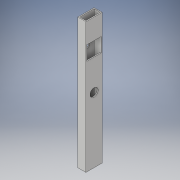
# Autodesk Inventor part: 2x1 16in Aluminum-ver2-1111-2020
Saved by Autodesk Inventor 2018 (Build 220112000, 112)
## iProperties
Created: 2020-01-28
Part Number: 2x1 16in Aluminum-ver2-1111-2020
Material: Generic
Document SubType Name: Modeling
Designer: JMHal
Density: 1 g/cm^3
Appearance: Default
Author: JMHal
Autodesk Inventor part; units mm, degrees
ref_plane "YZ Plane" through (0, 0, 0) normal (1, 0, 0) x (0, 1, 0)
ref_plane "XZ Plane" through (0, 0, 0) normal (0, 1, 0) x (-1, 0, 0)
ref_plane "XY Plane" through (0, 0, 0) normal (0, 0, 1) x (1, 0, 0)
sketch "Sketch1" plane through (0, 0, 0) normal (0, 1, 0) x (-1, 0, 0)
  line L0 (0, 0) -> (25.4, 0)
  line L1 (25.4, 0) -> (25.4, -50.8)
  line L2 (25.4, -50.8) -> (0, -50.8)
  line L3 (0, -50.8) -> (0, 0)
  line L4 (22.225, -47.625) -> (22.225, -3.175)
  line L5 (22.225, -3.175) -> (3.175, -3.175)
  line L6 (3.175, -3.175) -> (3.175, -47.625)
  line L7 (3.175, -47.625) -> (22.225, -47.625)
  dimension "d0" = 50.8
  dimension "d1" = 25.4
  dimension "d2" = 3.175
  constraints: 16 end point, 4 parallel, 2 perpendicular, 1 horizontal, 3 other
  measures "d0" distance between parallel lines of L2 L0
  measures "d1" distance between parallel lines of L1 L3
  measures "d2" distance between parallel lines of L1 L4
extrude "Extrusion1" add sketch "Sketch1" along normal blind 406.4
sketch "Sketch2" plane through (0, 0, 0) normal (1, 0, 0) x (0, 0, -1)
  circle A0 centre (25.4, 203.2) radius 12.7
  line L0 (0, 0) -> (0, 406.4) projected
  line L1 (50.8, 0) -> (0, 0) projected
  dimension "d5" = 25.4
  dimension "d6" = 25.4
  dimension "d7" = 203.2
  constraints: 1 centre point
  measures "d5" diameter of A0
  measures "d6" distance from line of A0.centre L0
  measures "d7" distance from line of A0.centre L1
extrude "Extrusion2" cut sketch "Sketch2" against normal blind 25.4
sketch "Sketch3" plane through (0, 0, 0) normal (1, 0, 0) x (0, 0, -1)
  line L0 (3.175, 0) -> (3.175, 406.4) projected
  line L1 (47.625, 0) -> (47.625, 406.4) projected
  line L2 (3.175, 342.9) -> (47.625, 342.9)
  line L3 (47.625, 342.9) -> (47.625, 298.45)
  line L4 (47.625, 298.45) -> (3.175, 298.45)
  line L5 (3.175, 298.45) -> (3.175, 342.9)
  line L6 (0, 406.4) -> (50.8, 406.4) projected
  point P0 (0, 0)
  dimension "d10" = 44.45
  dimension "d11" = 63.5
  constraints: 8 end point, 2 parallel, 2 point on line, 1 horizontal, 1 perpendicular
  measures "d10" distance between parallel lines of L4 L2
  measures "d11" distance between parallel lines of L6 L2
extrude "Extrusion3" cut sketch "Sketch3" against normal blind 12.7 contours L0 L2 L1 L4
sketch "Sketch4" plane through (-22.225, 0, -47.625) normal (1, 0, 0) x (0, 0, -1)
  circle A0 centre (-22.225, 317.5) radius 7.62
  line L0 (-47.625, 406.4) -> (3.175, 406.4) projected
  line L1 (-47.625, 0) -> (-47.625, 406.4) projected
  dimension "d14" = 88.9
  dimension "d15" = 25.4
  dimension "d16" = 15.24
  constraints: 1 centre point
  measures "d14" distance from line of L0 A0.centre
  measures "d15" distance from line of L1 A0.centre
  measures "d16" diameter of A0
extrude "Extrusion4" cut sketch "Sketch4" against normal blind 12.7
body "Solid1"
